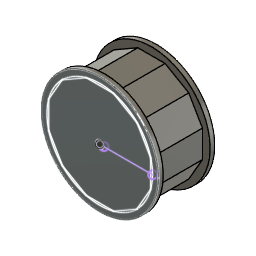
Wheel (Autodesk Fusion 360 design; units mm, degrees)
Autodesk Fusion 360 part; units mm, degrees
note: some values were not read from the file. Set by a fixed rule: which sketch regions a step uses.
sketch "Sketch1" plane through (0, 0, 0) normal (0, 0, 1) x (1, 0, 0)
  circle A0 centre (0, 0) radius 25
  circle A1 centre (0, 0) radius 22.5
  circle A2 centre (0, 0) radius 1.5
  line L0 (-0.912, -1.1909) -> (0.912, -1.1909)
  line L1 (5.8234, 21.7333) -> (-5.8234, 21.7333)
  line L2 (-5.8234, 21.7333) -> (-15.9099, 15.9099)
  line L3 (-15.9099, 15.9099) -> (-21.7333, 5.8234)
  line L4 (-21.7333, 5.8234) -> (-21.7333, -5.8234)
  line L5 (-21.7333, -5.8234) -> (-15.9099, -15.9099)
  line L6 (-15.9099, -15.9099) -> (-5.8234, -21.7333)
  line L7 (-5.8234, -21.7333) -> (5.8234, -21.7333)
  line L8 (5.8234, -21.7333) -> (15.9099, -15.9099)
  line L9 (15.9099, -15.9099) -> (21.7333, -5.8234)
  line L10 (21.7333, -5.8234) -> (21.7333, 5.8234)
  line L11 (21.7333, 5.8234) -> (15.9099, 15.9099)
  line L12 (15.9099, 15.9099) -> (5.8234, 21.7333)
  line L13 (1.75, 0) -> (22.5, 0)
  dimension "d2" = 50
  dimension "d3" = 45
  dimension "d4" = 3
  dimension "d5" = 1.824
  dimension "d38" = 2.5
  dimension "d42" = 22.5
  constraint coincident A0.centre A1.centre
  constraint concentric A1 A2
  constraint horizontal L0
  constraint coincident A2 L0.start
  constraint coincident A2 L0.end
  constraint parallel L1 L13
  measures "d2" diameter of A0
  measures "d3" diameter of A1
  measures "d4" diameter of A2
  measures "d5" distance of L0.start L0.end
  measures "d38" distance of A0 A1
  measures "d42" distance of L1.start A0.centre
extrude "Extrude6" add sketch "Sketch1" against normal blind 2 contours A0 | A1 L10 L13 | A1 L10 L13 | A1 L11 | L1 L2 L3 L4 L5 L6 L7 L8 L9 L10 L11 L12 | A1 L9 | A1 L12 | A1 L8 | A1 L1 | A1 L7 | A1 L2 | A1 L6 | A1 L3 | A1 L5 | A1 L4
extrude "Extrude7" add sketch "Sketch1" against normal blind 22 contours L1 L2 L3 L4 L5 L6 L7 L8 L9 L10 L11 L12
extrude "Extrude8" add sketch "Sketch1" along normal blind -24 and the other way blind 22 contours A0 | A1 L10 L13 | A1 L10 L13 | A1 L11 | L1 L2 L3 L4 L5 L6 L7 L8 L9 L10 L11 L12 | A1 L9 | A1 L12 | A1 L8 | A1 L1 | A1 L7 | A1 L2 | A1 L6 | A1 L3 | A1 L5 | A1 L4
equation "OuterDim = 50 mm"
equation "d2 = OuterDim"
equation "d3 = OuterDim * 0.9"
equation "Width = 20 mm"
equation "d42 = OuterDim * 0.9 / 2"
